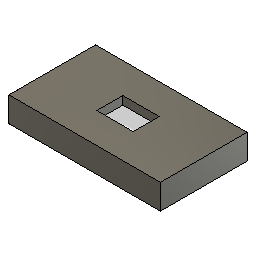
PPG Sleeve v2 (Autodesk Fusion 360 design; units mm, degrees)
Autodesk Fusion 360 part; units mm, degrees
sketch "Sketch1" plane through (0, 0, 0) normal (0, 1, 0) x (1, 0, 0)
  line L0 (0, 0) -> (25.9, 0)
  line L1 (25.9, 0) -> (25.9, 13.45)
  line L2 (25.9, 13.45) -> (0, 13.45)
  line L3 (0, 13.45) -> (0, 0)
  line L4 (-1.6, 15.05) -> (27.5, 15.05)
  line L5 (27.5, 15.05) -> (27.5, -1.6)
  line L6 (27.5, -1.6) -> (-1.6, -1.6)
  line L7 (-1.6, -1.6) -> (-1.6, 15.05)
  dimension "d1" = 25.9
  dimension "d2" = 13.45
  dimension "d3" = 1.6
  dimension "d4" = 1.6
  dimension "d5" = 1.6
  dimension "d6" = 1.6
  constraint horizontal L0
  constraint vertical L1
  constraint horizontal L2
  constraint vertical L3
  constraint coincident L0.start L3.end
  constraint horizontal L4
  constraint vertical L5
  constraint horizontal L6
  constraint vertical L7
  measures "d1" distance of L0.start L0.end
  measures "d2" distance of L0.start L2.end
  measures "d3" distance of L2 L4
  measures "d4" distance of L0 L6
  measures "d5" distance of L1 L5
  measures "d6" distance of L3 L7
extrude "Extrude1" add sketch "Sketch1" along normal blind 1.6 contours L0 L1 L2 L3 | L4 L5 L6 L7
extrude "Extrude2" add sketch "Sketch1" along normal blind 4.8
extrude "Extrude3" cut 1 faces at (0, 2.6667, -8.9667) along direction (-1, 0, 0) blind 1.6002
sketch "Sketch2" plane through (25.9, 0, 0) normal (-1, 0, 0) x (0, 0, 1)
  line L0 (-13.45, 1.6) -> (0, 1.6)
  line L1 (0, 1.6) -> (0, 4.8)
  line L2 (0, 4.8) -> (-13.45, 4.8)
  line L3 (-13.45, 4.8) -> (-13.45, 1.6)
  line L4 (-13.45, 4.8) -> (0, 4.8)
  line L5 (0, 4.8) -> (0, 3.2)
  line L6 (0, 3.2) -> (-13.45, 3.2)
  line L7 (-13.45, 3.2) -> (-13.45, 4.8)
  dimension "d13" = 1.6
  constraint horizontal L4
  constraint vertical L5
  constraint horizontal L6
  constraint vertical L7
  constraint coincident L2.end L3.start
  measures "d13" distance of L2.end L6.end
extrude "Extrude4" add sketch "Sketch2" along normal blind 27.5082 contours L1 L2 L3 L4 L5 L6 L7
sketch "Sketch3" plane through (0, 4.8, 0) normal (0, 1, 0) x (-1, 0, 0)
  line L0 (1.6, 0) -> (1.6, 1.6)
  line L1 (1.6, 1.6) -> (-27.5, 1.6)
  line L2 (-27.5, 1.6) -> (-27.5, -15.05)
  line L3 (-27.5, -15.05) -> (1.6, -15.05)
  line L4 (1.6, -15.05) -> (1.6, -13.45)
  line L5 (1.6, -13.45) -> (1.6082, -13.45)
  line L6 (1.6082, -13.45) -> (1.6082, 0)
  line L7 (1.6082, 0) -> (1.6, 0)
  line L8 (-9.4458, -9.2312) -> (-16.4458, -9.2312)
  line L9 (-16.4458, -9.2312) -> (-16.4458, -4.2312)
  line L10 (-16.4458, -4.2312) -> (-9.4458, -4.2312)
  line L11 (-9.4458, -4.2312) -> (-9.4458, -9.2312)
  line L12 (-9.4458, -9.2312) -> (-12.9458, -9.2312)
  line L13 (-12.9458, -9.2312) -> (-12.9458, -6.7312)
  line L14 (-12.9458, -6.7312) -> (-9.4458, -6.7312)
  line L15 (-9.4458, -6.7312) -> (-9.4458, -9.2312)
  dimension "d16" = 7
  dimension "d17" = 5
  dimension "d18" = 16.65
  dimension "d19" = 29.1
  dimension "d20" = 14.5542
  dimension "d21" = 8.3312
  constraint horizontal L8
  constraint vertical L9
  constraint horizontal L10
  constraint vertical L11
  constraint horizontal L12
  constraint vertical L13
  constraint horizontal L14
  constraint vertical L15
  measures "d16" distance of L8.start L8.end
  measures "d17" distance of L8.start L10.end
  measures "d18" distance of L1.end L2.end
  measures "d19" distance of L0.end L1.end
  measures "d20" distance of L2 L13.end
  measures "d21" distance of L1 L13.end
extrude "Extrude5" cut sketch "Sketch3" against normal blind 2.54 contours L8 L11 L12 L13 L14 L15 | L8 L9 L10 L11 L13 L14
extrude "Extrude6" cut 1 faces at (16.7333, 1.6, -4.4833) along direction (0, -1, 0) blind 0.8
sketch "Sketch4" plane through (-1.6, 0, 0) normal (-1, 0, 0) x (0, 0, 1)
  line L0 (0, 3.2) -> (0, 0.8)
  line L1 (0, 0.8) -> (-13.45, 0.8)
  line L2 (-13.45, 0.8) -> (-13.45, 3.2)
  line L3 (-13.45, 3.2) -> (-13.45, 4.8)
  line L4 (-13.45, 4.8) -> (-15.05, 4.8)
  line L5 (-15.05, 4.8) -> (-15.05, 0)
  line L6 (-15.05, 0) -> (1.6, 0)
  line L7 (1.6, 0) -> (1.6, 4.8)
  line L8 (1.6, 4.8) -> (0, 4.8)
  line L9 (0, 4.8) -> (0, 3.2)
  line L10 (-13.45, 0.8) -> (0, 0.8)
  line L11 (0, 0.8) -> (0, 0)
  line L12 (0, 0) -> (-13.45, 0)
  line L13 (-13.45, 0) -> (-13.45, 0.8)
  constraint horizontal L10
  constraint vertical L11
  constraint horizontal L12
  constraint vertical L13
  constraint coincident L11.end L12.start
  constraint coincident L1.end L2.start
extrude "Extrude7" cut sketch "Sketch4" against normal blind 27.5082 contours L1 L6 L10 L11 L12 L13
equation "d9 = 1.6 * 3 mm"
equation "d20 = ( 1.146 / 2 ) * 1 in"
equation "d21 = ( 0.656 / 2 ) * 1 in"
equation "d24 = -( 1.6 / 2 ) * 1 mm"
